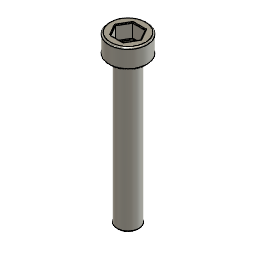
pcb_case (Autodesk Fusion 360 archive; units mm, degrees)
design "m3 x 20 mm"
Autodesk Fusion 360 part; units mm, degrees
sketch "Sketch1" plane through (0, 0, 0) normal (0, 1, 0) x (1, 0, 0)
  circle A0 centre (0, 0) radius 2.6
  circle A1 centre (0, 0) radius 1.5
  dimension "d1" = 5.2
  dimension "d2" = 3
  constraint coincident A0.centre A1.centre
  measures "d1" diameter of A0
  measures "d2" diameter of A1
extrude "Extrude1" add sketch "Sketch1" along normal blind 2.7 contours A0 | A1
extrude "Extrude2" add sketch "Sketch1" against normal blind 20 contours A1
sketch "Sketch2" plane through (0, 2.7, 0) normal (0, 1, 0) x (-1, 0, 0)
  circle A0 centre (0, 0) radius 2.6
  line L0 (0.866, -1.5) -> (1.7321, 0)
  line L1 (1.7321, 0) -> (0.866, 1.5)
  line L2 (0.866, 1.5) -> (-0.866, 1.5)
  line L3 (-0.866, 1.5) -> (-1.7321, 0)
  line L4 (-1.7321, 0) -> (-0.866, -1.5)
  line L5 (-0.866, -1.5) -> (0.866, -1.5)
  dimension "d7" = 1.5
  constraint coincident A0.centre origin
  measures "d7" distance of A0.centre L5
extrude "Extrude3" cut sketch "Sketch2" against normal blind 2 contours L0 L1 L2 L3 L4 L5
chamfer "Chamfer1" distance 0.1 angle 45 12 edges at (-1.299, 0.7, -0.75) (-1.299, 0.7, 0.75) (0, 0.7, 1.5) (1.299, 0.7, 0.75) (1.299, 0.7, -0.75) (1.299, 2.7, 0.75) (0, 2.7, 1.5) (-1.299, 2.7, 0.75) (-1.299, 2.7, -0.75) (0, 2.7, -1.5) (1.299, 2.7, -0.75) (0, 0.7, -1.5)
fillet "Fillet1" radius 0.2 4 edges at (-2.4241, 0, 0.9402) (-1.3985, -20, -0.5424) (-1.3985, 0, 0.5424) (-2.4241, 2.7, 0.9402)
equation "d7 = ( 3 / 2 ) * 1 mm"

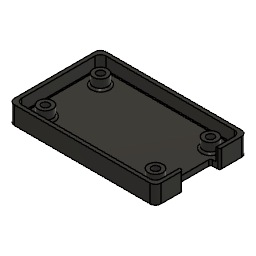
design "Bottom Housing"
Autodesk Fusion 360 part; units mm, degrees
sketch "base" plane through (0, 0, 0) normal (0, 1, 0) x (1, 0, 0)
  line L0 (0, 0) -> (80, 0) construction
  line L1 (80, 0) -> (80, 50) construction
  line L2 (80, 50) -> (0, 50) construction
  line L3 (0, 50) -> (0, 0) construction
  line L4 (0, 0) -> (5, 0)
  line L5 (5, 0) -> (5, 5) construction
  line L6 (5, 5) -> (75, 5) construction
  line L7 (75, 5) -> (75, 45) construction
  line L8 (75, 45) -> (5, 45) construction
  line L9 (5, 45) -> (5, 5) construction
  line L10 (5, 5) -> (10, 5) construction
  line L11 (10, 5) -> (10, 10) construction
  circle A0 centre (10, 10) radius 2
  line L12 (0, 25) -> (80, 25) construction
  line L13 (40, 0) -> (40, 50) construction
  circle A1 centre (10, 40) radius 2
  circle A2 centre (70, 40) radius 2
  circle A3 centre (70, 10) radius 2
  line L14 (0, 0) -> (80, 0)
  line L15 (80, 0) -> (80, 50)
  line L16 (80, 50) -> (0, 50)
  line L17 (0, 50) -> (0, 0)
  dimension "d1" = 80
  dimension "d2" = 50
  dimension "d3" = 5
  dimension "d4" = 5
  dimension "d5" = 70
  dimension "d6" = 40
  dimension "d7" = 5
  dimension "d8" = 5
  dimension "d9" = 4
  constraint horizontal L0
  constraint vertical L1
  constraint horizontal L2
  constraint vertical L3
  constraint coincident L0.start L3.end
  constraint perpendicular L3 L4
  constraint perpendicular L4 L5
  constraint horizontal L6
  constraint vertical L7
  constraint horizontal L8
  constraint vertical L9
  constraint perpendicular L9 L10
  constraint perpendicular L10 L11
  constraint coincident L11.end A0.centre
  constraint midpoint L3 L12.start
  constraint midpoint L1 L12.end
  constraint midpoint L0 L13.start
  constraint midpoint L2 L13.end
  constraint symmetric A0 L12 A1
  constraint symmetric A0 L13 A3
  constraint symmetric L13 A1 A2
  constraint horizontal L14
  constraint vertical L15
  constraint horizontal L16
  constraint vertical L17
  measures "d1" distance of L0.start L0.end
  measures "d2" distance of L0.start L2.end
  measures "d3" distance of L0.start L4.end
  measures "d4" distance of L4.end L5.end
  measures "d5" distance of L5.end L6.end
  measures "d6" distance of L5.end L8.end
  measures "d7" distance of L5.end L10.end
  measures "d8" distance of L10.end L11.end
  measures "d9" diameter of A0
extrude "Extrude1" add sketch "base" along normal blind 10
sketch "cutout_standoffs" plane through (0, 10, 0) normal (0, 1, 0) x (-1, 0, 0)
  circle A0 centre (-70, -40) radius 2
  circle A1 centre (-10, -10) radius 2
  circle A2 centre (-10, -40) radius 2
  circle A3 centre (-70, -10) radius 2
  line L0 (0, -50) -> (0, 0)
  line L1 (0, 0) -> (-80, 0)
  line L2 (-80, 0) -> (-80, -50)
  line L3 (-80, -50) -> (0, -50)
  line L4 (0, 0) -> (-80, 0)
  line L5 (-80, 0) -> (-80, -50)
  line L6 (-80, -50) -> (0, -50)
  line L7 (0, -50) -> (0, 0)
  line L8 (0, 0) -> (-2, 0)
  line L9 (-2, 0) -> (-2, -2)
  line L10 (-2, -2) -> (-78, -2)
  line L11 (-78, -2) -> (-78, -48)
  line L12 (-78, -48) -> (-2, -48)
  line L13 (-2, -48) -> (-2, -2)
  circle A4 centre (-10, -40) radius 4
  circle A5 centre (-70, -40) radius 4
  circle A6 centre (-10, -10) radius 4
  circle A7 centre (-70, -10) radius 4
  dimension "d12" = 2
  dimension "d13" = 2
  dimension "d14" = 76
  dimension "d15" = 46
  dimension "d16" = 8
  dimension "d17" = 8
  dimension "d18" = 8
  dimension "d19" = 8
  constraint horizontal L4
  constraint vertical L5
  constraint horizontal L6
  constraint vertical L7
  constraint coincident L2.end L3.start
  constraint coincident L0.end L1.start
  constraint coincident L1 L8.end
  constraint perpendicular L1 L9
  constraint horizontal L10
  constraint vertical L11
  constraint horizontal L12
  constraint vertical L13
  constraint concentric A2 A4
  constraint concentric A0 A5
  constraint concentric A1 A6
  constraint concentric A3 A7
  measures "d12" distance of L0.end L8.end
  measures "d13" distance of L8.end L9.end
  measures "d14" distance of L9.end L10.end
  measures "d15" distance of L9.end L12.end
  measures "d16" diameter of A4
  measures "d17" diameter of A5
  measures "d18" diameter of A6
  measures "d19" diameter of A7
extrude "Extrude2" cut sketch "cutout_standoffs" against normal blind 7 contours L10 L11 L12 L13
extrude "Extrude3" cut 4 faces at (6.689, 10, -40.2981) (6.689, 10, -10.2981) (66.6816, 10, -10.1987) (66.6816, 10, -40.1987) along direction (0, -1, 0) blind 1.6
fillet "Fillet1" radius 3 8 edges at (78, 6.5, -2) (78, 6.5, -48) (2, 6.5, -48) (2, 6.5, -2) (0, 5, -50) (0, 5, 0) (80, 5, -50) (80, 5, 0)
chamfer "Chamfer1" distance 1 angle 45 4 edges at (73.7293, 3, -11.4465) (73.7293, 3, -41.4465) (13.7293, 3, -41.4465) (13.7293, 3, -11.4465)
sketch "cutout_rj45" plane through (80, 0, 0) normal (1, 0, 0) x (0, 0, -1)
  line L0 (3, 10) -> (3, 0)
  line L1 (3, 0) -> (47, 0)
  line L2 (47, 0) -> (47, 10)
  line L3 (47, 10) -> (3, 10)
  line L4 (25, 0) -> (25, 10) construction
  line L5 (25, 10) -> (25, 0) construction
  line L6 (25, 0) -> (15, 0)
  line L7 (15, 0) -> (15, 10)
  line L8 (35, 0) -> (35, 10)
  line L9 (25, 0) -> (35, 0)
  dimension "d27" = 10
  dimension "d28" = 10
  constraint midpoint L1 L4.start
  constraint midpoint L3 L4.end
  constraint perpendicular L3 L5
  constraint perpendicular L0 L6
  constraint coincident L3 L7.end
  constraint perpendicular L3 L7
  constraint symmetric L4 L5.end L6.start
  constraint symmetric L4 L6.end L8.start
  constraint symmetric L4 L7.end L8.end
  measures "d27" distance of L4.end L4.start
  measures "d28" distance of L4.start L6.end
extrude "Extrude4" cut sketch "cutout_rj45" against normal blind 5 contours L1 L3 L6 L7 L8 L9
chamfer "Chamfer2" distance 0.2 angle 45 9 edges at (40, 0, 0) (79.1213, 0, -0.8787) (80, 0, -9) (80, 0, -41) (79.1213, 0, -49.1213) (40, 0, -50) (0.8787, 0, -49.1213) (0, 0, -25) (0.8787, 0, -0.8787)
fillet "Fillet3" radius 0.4 9 edges at (77.1213, 3, -47.1213) (78, 3, -10) (78, 3, -40) (77.1213, 3, -2.8787) (40, 3, -2) (2.8787, 3, -2.8787) (2, 3, -25) (2.8787, 3, -47.1213) (40, 3, -48)
fillet "Fillet4" radius 1 4 edges at (75, 1.5, -15) (75, 1.5, -35) (80, 5.1, -35) (80, 5.1, -15)
equation "d1 = 70 mm + 10 mm"
equation "d2 = 40 mm + 10 mm"

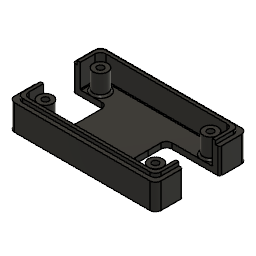
design "Top Housing"
Autodesk Fusion 360 part; units mm, degrees
sketch "base" plane through (0, 0, 0) normal (0, 1, 0) x (1, 0, 0)
  line L0 (0, 0) -> (80, 0) construction
  line L1 (80, 0) -> (80, 50) construction
  line L2 (80, 50) -> (0, 50) construction
  line L3 (0, 50) -> (0, 0) construction
  line L4 (0, 0) -> (5, 0)
  line L5 (5, 0) -> (5, 5) construction
  line L6 (5, 5) -> (75, 5) construction
  line L7 (75, 5) -> (75, 45) construction
  line L8 (75, 45) -> (5, 45) construction
  line L9 (5, 45) -> (5, 5) construction
  line L10 (5, 5) -> (10, 5) construction
  line L11 (10, 5) -> (10, 10) construction
  circle A0 centre (10, 10) radius 1.75
  line L12 (0, 25) -> (80, 25) construction
  line L13 (40, 0) -> (40, 50) construction
  circle A1 centre (10, 40) radius 1.75
  circle A2 centre (70, 40) radius 1.75
  circle A3 centre (70, 10) radius 1.75
  line L14 (0, 0) -> (80, 0)
  line L15 (80, 0) -> (80, 50)
  line L16 (80, 50) -> (0, 50)
  line L17 (0, 50) -> (0, 0)
  dimension "d1" = 80
  dimension "d2" = 50
  dimension "d3" = 5
  dimension "d4" = 5
  dimension "d5" = 70
  dimension "d6" = 40
  dimension "d7" = 5
  dimension "d8" = 5
  dimension "d9" = 3.5
  constraint horizontal L0
  constraint vertical L1
  constraint horizontal L2
  constraint vertical L3
  constraint coincident L0.start L3.end
  constraint perpendicular L3 L4
  constraint perpendicular L4 L5
  constraint horizontal L6
  constraint vertical L7
  constraint horizontal L8
  constraint vertical L9
  constraint perpendicular L9 L10
  constraint perpendicular L10 L11
  constraint coincident L11.end A0.centre
  constraint midpoint L3 L12.start
  constraint midpoint L1 L12.end
  constraint midpoint L0 L13.start
  constraint midpoint L2 L13.end
  constraint symmetric A0 L12 A1
  constraint symmetric A0 L13 A3
  constraint symmetric L13 A1 A2
  constraint horizontal L14
  constraint vertical L15
  constraint horizontal L16
  constraint vertical L17
  measures "d1" distance of L0.start L0.end
  measures "d2" distance of L0.start L2.end
  measures "d3" distance of L0.start L4.end
  measures "d4" distance of L4.end L5.end
  measures "d5" distance of L5.end L6.end
  measures "d6" distance of L5.end L8.end
  measures "d7" distance of L5.end L10.end
  measures "d8" distance of L10.end L11.end
  measures "d9" diameter of A0
extrude "Extrude1" add sketch "base" along normal blind 10
sketch "inter_base" plane through (0, 10, 0) normal (0, 1, 0) x (-1, 0, 0)
  circle A0 centre (-70, -40) radius 1.75
  circle A1 centre (-10, -10) radius 1.75
  circle A2 centre (-10, -40) radius 1.75
  circle A3 centre (-70, -10) radius 1.75
  line L0 (0, -50) -> (0, 0)
  line L1 (0, 0) -> (-80, 0)
  line L2 (-80, 0) -> (-80, -50)
  line L3 (-80, -50) -> (0, -50)
  line L4 (0, 0) -> (-80, 0)
  line L5 (-80, 0) -> (-80, -50)
  line L6 (-80, -50) -> (0, -50)
  line L7 (0, -50) -> (0, 0)
  line L8 (0, 0) -> (-4, 0)
  line L9 (-4, 0) -> (-4, -4)
  line L10 (-4, -4) -> (-76, -4)
  line L11 (-76, -4) -> (-76, -46)
  line L12 (-76, -46) -> (-4, -46)
  line L13 (-4, -46) -> (-4, -4)
  circle A4 centre (-10, -40) radius 4
  circle A5 centre (-70, -40) radius 4
  circle A6 centre (-10, -10) radius 4
  circle A7 centre (-70, -10) radius 4
  line L14 (0, -25) -> (-80, -25) construction
  line L15 (-40, -50) -> (-40, 0) construction
  dimension "d12" = 4
  dimension "d13" = 4
  dimension "d14" = 72
  dimension "d15" = 42
  dimension "d16" = 8
  dimension "d17" = 8
  dimension "d18" = 8
  dimension "d19" = 8
  constraint horizontal L4
  constraint vertical L5
  constraint horizontal L6
  constraint vertical L7
  constraint coincident L2.end L3.start
  constraint coincident L0.end L1.start
  constraint coincident L1 L8.end
  constraint perpendicular L1 L9
  constraint horizontal L10
  constraint vertical L11
  constraint horizontal L12
  constraint vertical L13
  constraint concentric A2 A4
  constraint concentric A0 A5
  constraint concentric A1 A6
  constraint concentric A3 A7
  constraint midpoint L7 L14.start
  constraint midpoint L5 L14.end
  constraint midpoint L3 L15.start
  constraint midpoint L4 L15.end
  measures "d12" distance of L0.end L8.end
  measures "d13" distance of L8.end L9.end
  measures "d14" distance of L9.end L10.end
  measures "d15" distance of L9.end L12.end
  measures "d16" diameter of A4
  measures "d17" diameter of A5
  measures "d18" diameter of A6
  measures "d19" diameter of A7
extrude "Extrude2" cut sketch "inter_base" against normal blind 7 contours L10 L11 L12 L13
extrude "Extrude3" cut 4 faces at (6.7714, 10, -40.2857) (6.7714, 10, -10.2857) (66.7649, 10, -10.1987) (66.7649, 10, -40.1987) along direction (0, -1, 0) blind 2
fillet "Fillet1" radius 3 8 edges at (76, 6.5, -4) (76, 6.5, -46) (4, 6.5, -46) (4, 6.5, -4) (0, 5, -50) (0, 5, 0) (80, 5, -50) (80, 5, 0)
chamfer "Chamfer1" distance 1 angle 45 4 edges at (73.7293, 3, -11.4465) (73.7293, 3, -41.4465) (13.7293, 3, -41.4465) (13.7293, 3, -11.4465)
extrude "Extrude5" cut 1 faces at (29, 10, -1.3333) along direction (0, -1, 0) blind 2
extrude "Extrude6" add 5 faces at (6.7714, 8, -10.2857) (29, 8, -1.3333) (6.7714, 8, -40.2857) (66.7649, 8, -10.1987) (66.7649, 8, -40.1987) along direction (0, 1, 0) blind 6
chamfer "Chamfer2" distance 0.4 angle 45 4 edges at (68.3684, 0, -10.6328) (8.3684, 0, -10.6328) (8.3684, 0, -40.6328) (68.3684, 0, -40.6328)
sketch "top" plane through (0, 0, 0) normal (0, -1, 0) x (1, 0, 0)
  circle A0 centre (10, -40) radius 2.15
  circle A1 centre (70, -10) radius 2.15
  arc A2 (80, -3) -> (77, 0) centre (77, -3) ccw
  line L0 (77, 0) -> (3, 0)
  arc A3 (3, 0) -> (0, -3) centre (3, -3) ccw
  line L1 (0, -3) -> (0, -47)
  arc A4 (0, -47) -> (3, -50) centre (3, -47) ccw
  line L2 (3, -50) -> (77, -50)
  arc A5 (77, -50) -> (80, -47) centre (77, -47) ccw
  line L3 (80, -47) -> (80, -3)
  circle A6 centre (10, -10) radius 2.15
  circle A7 centre (70, -40) radius 2.15
  line L4 (0, -25) -> (80, -25) construction
  line L5 (0, -25) -> (0, -15)
  line L6 (40, -25) -> (40, 0) construction
  line L7 (80, -15) -> (50.923, -15)
  line L8 (50.923, -15) -> (50.9933, -25)
  line L9 (50.9933, -35) -> (50.9933, -24.8594)
  line L10 (80, -35) -> (50.9933, -35)
  line L11 (18.75, -15) -> (18.75, -35)
  line L12 (18.75, -35) -> (0, -35)
  line L13 (18.75, -15) -> (0, -15)
  dimension "d38" = 10
  constraint midpoint L1 L4.start
  constraint midpoint L3 L4.end
  constraint perpendicular L4 L5
  constraint midpoint L4 L6.start
  constraint midpoint L0 L6.end
  constraint symmetric L5.end L6 L7.start
  constraint coincident L1 L12.end
  constraint perpendicular L1 L12
  constraint perpendicular L1 L13
  constraint coincident L8.end L9
  constraint coincident L4 L8.end
  measures "d38" distance of L4.start L5.end
extrude "Extrude7" cut sketch "top" against normal blind 18 contours L3 L7 L8 L9 L10 | L1 L5 L11 L12 L13
fillet "Fillet3" radius 3 4 edges at (18.75, 1.5, -35) (18.75, 1.5, -15) (50.9933, 1.5, -35) (50.923, 1.5, -15)
sketch "inter_edge_z-" plane through (0, 14, 0) normal (0, 1, 0) x (-1, 0, 0)
  line L0 (0, -35) -> (-4, -35)
  line L1 (-4, -35) -> (-4, -43)
  arc A0 (-7, -46) -> (-4, -43) centre (-7, -43) ccw
  line L2 (-7, -46) -> (-73, -46)
  arc A1 (-76, -43) -> (-73, -46) centre (-73, -43) ccw
  line L3 (-76, -43) -> (-76, -35)
  line L4 (-76, -35) -> (-80, -35)
  line L5 (-80, -35) -> (-80, -47)
  arc A2 (-80, -47) -> (-77, -50) centre (-77, -47) ccw
  line L6 (-77, -50) -> (-3, -50)
  arc A3 (-3, -50) -> (0, -47) centre (-3, -47) ccw
  line L7 (0, -47) -> (0, -35)
  line L8 (-4, -35) -> (-2.25, -35)
  line L9 (-2.25, -35) -> (-2.25, -43)
  line L10 (-7, -46) -> (-7, -47.75) construction
  line L11 (-2.25, -43) -> (-2.25, -47.75)
  line L12 (-2.25, -47.75) -> (-7, -47.75)
  line L13 (-7, -47.75) -> (-76, -47.75)
  line L14 (-76, -47.75) -> (-77.75, -47.75)
  line L15 (-77.75, -47.75) -> (-77.75, -34.99)
  dimension "d49" = 1.75
  dimension "d50" = 1.75
  dimension "d51" = 1.75
  constraint coincident L0.end L1.start
  constraint perpendicular L1 L8
  constraint perpendicular L0 L9
  constraint coincident A0.start L2.start
  constraint perpendicular L2 L10
  constraint parallel L10 L11
  constraint perpendicular L10 L12
  constraint perpendicular L3 L13
  constraint parallel L13 L14
  constraint vertical L15
  measures "d49" distance of L0.end L8.end
  measures "d50" distance of A0.start L10.end
  measures "d51" distance of L13.end L14.end
extrude "Extrude9" add sketch "inter_edge_z-" along normal blind 2 contours L0 L1 A0 L2 A1 L3 L4 L8 L9 L11 L12 L13 L14 L15
fillet "Fillet5" radius 3 2 edges at (2.25, 15, -47.75) (77.75, 15, -47.75)
sketch "inter_edge_z+" plane through (0, 14, 0) normal (0, 1, 0) x (-1, 0, 0)
  line L0 (-4, -15) -> (0, -15)
  line L1 (0, -15) -> (0, -3)
  arc A0 (0, -3) -> (-3, 0) centre (-3, -3) ccw
  line L2 (-3, 0) -> (-77, 0)
  arc A1 (-77, 0) -> (-80, -3) centre (-77, -3) ccw
  line L3 (-80, -3) -> (-80, -15)
  line L4 (-80, -15) -> (-76, -15)
  line L5 (-76, -15) -> (-76, -7)
  arc A2 (-73, -4) -> (-76, -7) centre (-73, -7) ccw
  line L6 (-73, -4) -> (-7, -4)
  arc A3 (-4, -7) -> (-7, -4) centre (-7, -7) ccw
  line L7 (-4, -7) -> (-4, -15)
  line L8 (-4, -15) -> (-2.25, -15)
  line L9 (-7, -4) -> (-7, -2.25) construction
  line L10 (-2.25, -15) -> (-2.25, -2.25)
  line L11 (-2.25, -2.25) -> (-7, -2.25)
  line L12 (-76, -15) -> (-77.75, -15)
  line L13 (-73, -4) -> (-73, -2.25) construction
  line L14 (-77.75, -15) -> (-77.75, -2.25)
  line L15 (-77.75, -2.25) -> (-7, -2.25)
  dimension "d56" = 1.75
  dimension "d57" = 1.75
  dimension "d58" = 1.75
  dimension "d59" = 1.75
  constraint coincident L0.start L7.end
  constraint perpendicular L7 L8
  constraint coincident L6.end A3.end
  constraint perpendicular L6 L9
  constraint perpendicular L0 L10
  constraint perpendicular L9 L11
  constraint coincident L4.end L5.start
  constraint perpendicular L5 L12
  constraint coincident A2.start L6.start
  constraint perpendicular L6 L13
  constraint perpendicular L4 L14
  constraint perpendicular L14 L15
  measures "d56" distance of L0.start L8.end
  measures "d57" distance of L6.end L9.end
  measures "d58" distance of L4.end L12.end
  measures "d59" distance of A2.start L13.end
extrude "Extrude10" add sketch "inter_edge_z+" along normal blind 2 contours L0 L4 L5 A2 L6 A3 L7 L8 L10 L11 L12 L14 L15
fillet "Fillet6" radius 3 2 edges at (2.25, 15, -2.25) (77.75, 15, -2.25)
fillet "Fillet7" radius 0.4 10 edges at (4, 3, -39) (4.8787, 3, -45.1213) (40, 3, -46) (75.1213, 3, -45.1213) (76, 3, -39) (76, 3, -11) (75.1213, 3, -4.8787) (40, 3, -4) (4.8787, 3, -4.8787) (4, 3, -11)
fillet "Fillet8" radius 1 4 edges at (80, 7, -15) (80, 7, -35) (0, 7, -35) (0, 7, -15)
equation "d1 = 70 mm + 10 mm"
equation "d2 = 40 mm + 10 mm"

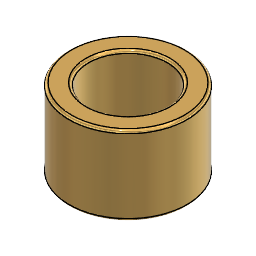
design "m3_brass_inserts"
Autodesk Fusion 360 part; units mm, degrees
sketch "Sketch1" plane through (0, 0, 0) normal (0, 1, 0) x (1, 0, 0)
  circle A0 centre (0, 0) radius 2.25
  circle A1 centre (0, 0) radius 1.5
  dimension "d1" = 4.5
  dimension "d2" = 3
  constraint coincident A0.centre A1.centre
  constraint concentric A0 A1
  measures "d1" diameter of A0
  measures "d2" diameter of A1
extrude "Extrude1" add sketch "Sketch1" along normal blind 3
fillet "Fillet1" radius 0.1 4 edges at (-2.0977, 0, 0.8136) (-1.3985, 0, -0.5424) (-1.3985, 3, -0.5424) (-2.0977, 3, 0.8136)
